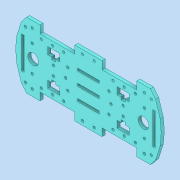
# Autodesk Inventor part: 底盘设计2.0
Saved by Autodesk Inventor 2019 (Build 230136000, 136)
## iProperties
Created: 2020-10-19
Part Number: 底盘设计2.0
Material: 乙缩醛树脂，白色
Document SubType Name: Modeling
Designer: Wang Hua
Density: 1.425 g/cm^3
Appearance: 平滑 - 白色
Author: Wang Hua
Autodesk Inventor part; units mm, degrees
ref_plane "YZ Plane" through (0, 0, 0) normal (1, 0, 0) x (0, 1, 0)
ref_plane "XZ Plane" through (0, 0, 0) normal (0, 1, 0) x (-1, 0, 0)
ref_plane "XY Plane" through (0, 0, 0) normal (0, 0, 1) x (1, 0, 0)
sketch "草图1" plane through (0, 0, 0) normal (0, 0, 1) x (1, 0, 0)
  line L0 (-80, -42.5) -> (-80, -32.5) construction
  line L1 (80, -42.5) -> (-80, 42.5) construction
  line L2 (-80, -42.5) -> (80, 42.5) construction
  line L3 (-17.5754, 32.5) -> (-62.5754, 32.5)
  line L4 (-62.5754, 32.5) -> (-62.5754, 42.5)
  line L5 (-17.5754, 42.5) -> (-17.5754, 32.5)
  line L6 (0, 0) -> (0, 68.1065) construction
  line L7 (0, 0) -> (-105.3921, 0) construction
  line L8 (17.5754, 32.5) -> (62.5754, 32.5)
  line L9 (62.5754, 32.5) -> (62.5754, 42.5)
  line L10 (17.5754, 42.5) -> (17.5754, 32.5)
  line L11 (-17.5754, -32.5) -> (-62.5754, -32.5)
  line L12 (-62.5754, -32.5) -> (-62.5754, -42.5)
  line L13 (-17.5754, -42.5) -> (-17.5754, -32.5)
  line L14 (62.5754, -32.5) -> (62.5754, -42.5)
  line L15 (17.5754, -32.5) -> (62.5754, -32.5)
  line L16 (17.5754, -42.5) -> (17.5754, -32.5)
  line L17 (-80, 42.5) -> (-62.5754, 42.5)
  line L18 (-17.5754, 42.5) -> (17.5754, 42.5)
  line L19 (62.5754, 42.5) -> (80, 42.5)
  line L20 (80, -42.5) -> (62.5754, -42.5)
  line L21 (17.5754, -42.5) -> (-17.5754, -42.5)
  line L22 (-62.5754, -42.5) -> (-80, -42.5)
  arc A0 (-92.6213, 15.4186) -> (-92.6213, -15.4186) centre (4.8977, 0) ccw
  line L23 (-80, 42.5) -> (-86.7375, 34.0532)
  line L24 (-86.7375, 34.0532) -> (-92.6213, 15.4186)
  line L25 (-80, -42.5) -> (-86.7375, -34.0532)
  line L26 (-86.7375, -34.0532) -> (-92.6213, -15.4186)
  arc A1 (92.6213, -15.4186) -> (92.6213, 15.4186) centre (-4.8977, 0) ccw
  line L27 (80, 42.5) -> (86.7375, 34.0532)
  line L28 (86.7375, 34.0532) -> (92.6213, 15.4186)
  line L29 (80, -42.5) -> (86.7375, -34.0532)
  line L30 (86.7375, -34.0532) -> (92.6213, -15.4186)
  line L31 (80, 42.5) -> (80, 32.5) construction
  circle A2 centre (-71.2877, 0) radius 7
  line L32 (-83.1946, -20.7208) -> (-86.3946, -20.7208)
  line L33 (-86.3946, -20.7208) -> (-86.3946, 20.7208)
  line L34 (-86.3946, 20.7208) -> (-83.1946, 20.7208)
  line L35 (-83.1946, 20.7208) -> (-83.1946, -20.7208)
  line L36 (-83.1946, -20.7208) -> (-86.3946, 20.7208) construction
  line L37 (-86.3946, -20.7208) -> (-83.1946, 20.7208) construction
  line L38 (-35.0754, 53.2522) -> (-35.0754, 15.4186) construction
  line L39 (-52.6567, 14.2921) -> (-52.6567, 23.3874)
  line L40 (-52.6567, 23.3874) -> (-36.8922, 23.3874)
  line L41 (-36.8922, 23.3874) -> (-36.8922, 14.2921)
  line L42 (-27.1931, 14.2921) -> (-42.9577, 23.3874) construction
  line L43 (-42.9577, 14.2921) -> (-27.1931, 23.3874) construction
  line L44 (-42.2559, 11.1975) -> (-47.2929, 11.1975)
  line L45 (-47.2929, 11.1975) -> (-47.2929, 14.2921)
  line L46 (-42.2559, 14.2921) -> (-42.2559, 11.1975)
  line L47 (-32.5569, 11.1975) -> (-37.5939, 17.3867) construction
  line L48 (-37.5939, 11.1975) -> (-32.5569, 17.3867) construction
  line L49 (-36.8922, 14.2921) -> (-42.2559, 14.2921)
  line L50 (-47.2929, 14.2921) -> (-52.6567, 14.2921)
  line L51 (-14.0581, 18.6186) -> (14.0581, 18.6186)
  line L52 (14.0581, 18.6186) -> (14.0581, 15.4186)
  line L53 (14.0581, 15.4186) -> (-14.0581, 15.4186)
  line L54 (-14.0581, 15.4186) -> (-14.0581, 18.6186)
  line L55 (14.0581, -1.6) -> (-14.0581, -1.6)
  line L56 (-14.0581, -1.6) -> (-14.0581, 1.6)
  line L57 (-14.0581, 1.6) -> (14.0581, 1.6)
  line L58 (14.0581, 1.6) -> (14.0581, -1.6)
  line L59 (14.0581, -1.6) -> (-14.0581, 1.6) construction
  line L60 (-14.0581, -1.6) -> (14.0581, 1.6) construction
  line L61 (-52.6567, -14.2921) -> (-52.6567, -23.3874)
  line L62 (-52.6567, -23.3874) -> (-36.8922, -23.3874)
  line L63 (-36.8922, -23.3874) -> (-36.8922, -14.2921)
  line L64 (-42.2559, -11.1975) -> (-47.2929, -11.1975)
  line L65 (-47.2929, -11.1975) -> (-47.2929, -14.2921)
  line L66 (-42.2559, -14.2921) -> (-42.2559, -11.1975)
  line L67 (-36.8922, -14.2921) -> (-42.2559, -14.2921)
  line L68 (-47.2929, -14.2921) -> (-52.6567, -14.2921)
  line L69 (-14.0581, -18.6186) -> (14.0581, -18.6186)
  line L70 (14.0581, -18.6186) -> (14.0581, -15.4186)
  line L71 (14.0581, -15.4186) -> (-14.0581, -15.4186)
  line L72 (-14.0581, -15.4186) -> (-14.0581, -18.6186)
  line L73 (80, -42.5) -> (80, -32.5) construction
  line L74 (52.6567, 14.2921) -> (52.6567, 23.3874)
  line L75 (52.6567, 23.3874) -> (36.8922, 23.3874)
  line L76 (36.8922, 23.3874) -> (36.8922, 14.2921)
  line L77 (42.2559, 11.1975) -> (47.2929, 11.1975)
  line L78 (47.2929, 11.1975) -> (47.2929, 14.2921)
  line L79 (42.2559, 14.2921) -> (42.2559, 11.1975)
  line L80 (36.8922, 14.2921) -> (42.2559, 14.2921)
  line L81 (47.2929, 14.2921) -> (52.6567, 14.2921)
  line L82 (36.8922, -23.3874) -> (36.8922, -14.2921)
  line L83 (52.6567, -23.3874) -> (36.8922, -23.3874)
  line L84 (52.6567, -14.2921) -> (52.6567, -23.3874)
  line L85 (47.2929, -14.2921) -> (52.6567, -14.2921)
  line L86 (47.2929, -11.1975) -> (47.2929, -14.2921)
  line L87 (42.2559, -11.1975) -> (47.2929, -11.1975)
  line L88 (42.2559, -14.2921) -> (42.2559, -11.1975)
  line L89 (36.8922, -14.2921) -> (42.2559, -14.2921)
  circle A3 centre (71.2877, 0) radius 7
  line L90 (83.1946, -20.7208) -> (86.3946, -20.7208)
  line L91 (86.3946, -20.7208) -> (86.3946, 20.7208)
  line L92 (86.3946, 20.7208) -> (83.1946, 20.7208)
  line L93 (83.1946, 20.7208) -> (83.1946, -20.7208)
  line L94 (86.3946, -20.7208) -> (83.1946, 20.7208) construction
  line L95 (0, 0) -> (51.2908, 0) construction
  point P0 (-84.7946, 0)
  point P1 (7.5, 37.2039)
  point P2 (-7.5, 37.2039)
  point P3 (-21.5, 37.1159)
  point P4 (21.5, 37.1159)
  point P5 (-35.0754, 18.8397)
  point P6 (-45.0754, 6.0335)
  point P7 (7.5, -37.2039)
  point P8 (-7.5, -37.2039)
  point P9 (-21.5, -37.1159)
  point P10 (21.5, -37.1159)
  point P11 (-45.0754, -6.0335)
  point P12 (-29.2838, 0)
  point P13 (-26.6075, 13)
  point P14 (-26.6075, -13)
  point P15 (45.0754, 6.0335)
  point P16 (45.0754, -6.0335)
  point P17 (29.2838, 0)
  point P18 (26.6075, 13)
  point P19 (26.6075, -13)
  point P20 (-81.3188, 31.1796)
  point P21 (-81.3188, -31.1796)
  point P22 (81.3188, 31.1796)
  point P23 (81.3188, -31.1796)
  point P24 (60.8153, 27.4236)
  point P25 (46.3153, 27.4236)
  point P26 (31.8153, 27.4236)
  point P27 (60.8153, -27.4236)
  point P28 (46.3153, -27.4236)
  point P29 (31.8153, -27.4236)
  point P30 (-60.8153, 27.4236)
  point P31 (-46.3153, 27.4236)
  point P32 (-31.8153, 27.4236)
  point P33 (-46.3153, -27.4236)
  point P34 (-60.8153, -27.4236)
  point P35 (-31.8153, -27.4236)
  point P36 (72.4718, 34.0532)
  point P37 (72.4718, 17.0686)
  point P38 (72.4718, -34.0532)
  point P39 (72.4718, -17.0686)
  point P40 (-72.4718, 34.0532)
  point P41 (-72.4718, 17.0686)
  point P42 (-72.4718, -17.0686)
  point P43 (-72.4718, -34.0532)
  point P44 (-40.0754, 32.5)
  point P45 (40.0754, 32.5)
  dimension "d0" = 160
  dimension "d1" = 85
  dimension "d2" = 10
  dimension "d3" = 45
  dimension "d4" = 14
  dimension "d5" = 3.2
  dimension "d6" = 7.5
  dimension "d7" = 14
  dimension "d8" = 17.5
  dimension "d9" = 3.2
  dimension "d10" = 3.2
  dimension "d11" = 13
  dimension "d16" = 14.5
  dimension "d17" = 14.5
  constraints: 192 end point, 68 symmetric about line, 21 parallel, 12 horizontal, 10 midpoint, 10 perpendicular, 7 point on line, 4 centre point, 4 point on circle, 2 vertical, 5 other
  measures "d0" distance of L2.end L1.end
  measures "d1" distance of L0.start L1.end
  measures "d2" distance of L12.start L12.end
  measures "d3" distance of L3.start L3.end
  measures "d4" diameter of A2
  measures "d5" distance of L34.end L33.end
  measures "d6" distance from line of point (7.5, 37.204) L6
  measures "d7" horizontal distance of point (21.5, 37.116) point (7.5, 37.204)
  measures "d8" distance between parallel lines of L5 L38
  measures "d9" distance of L53.end L51.start
  measures "d10" distance of L55.end L56.end
  measures "d11" distance from line of L7 point (-26.608, 13)
  measures "d16" distance of point (46.315, 27.424) point (60.815, 27.424)
  measures "d17" distance of point (31.815, 27.424) point (46.315, 27.424)
extrude "拉伸1" add sketch "草图1" along normal blind 4
hole "孔1" at (7.5, 37.2039, 0) at (-7.5, 37.2039, 0) at (-21.5, 37.1159, 0) at (21.5, 37.1159, 0) at (-45.0754, 6.0335, 0) at (21.5, -37.1159, 0) at (7.5, -37.2039, 0) at (-7.5, -37.2039, 0) at (-21.5, -37.1159, 0) at (-45.0754, -6.0335, 0) at (-29.2838, 0, 0) at (-26.6075, 13, 0) at (-26.6075, -13, 0) at (45.0754, 6.0335, 0) at (45.0754, -6.0335, 0) at (29.2838, 0, 0) at (26.6075, 13, 0) at (26.6075, -13, 0) at (-81.3188, 31.1796, 0) at (-81.3188, -31.1796, 0) at (81.3188, 31.1796, 0) at (81.3188, -31.1796, 0) at (60.8153, 27.4236, 0) at (46.3153, 27.4236, 0) at (31.8153, 27.4236, 0) at (46.3153, -27.4236, 0) at (60.8153, -27.4236, 0) at (31.8153, -27.4236, 0) at (-60.8153, 27.4236, 0) at (-46.3153, 27.4236, 0) at (-31.8153, 27.4236, 0) at (-60.8153, -27.4236, 0) at (-46.3153, -27.4236, 0) at (-31.8153, -27.4236, 0) at (72.4718, 34.0532, 0) at (72.4718, 17.0686, 0) at (72.4718, -17.0686, 0) at (72.4718, -34.0532, 0) at (-72.4718, 34.0532, 0) at (-72.4718, 17.0686, 0) at (-72.4718, -17.0686, 0) at (-72.4718, -34.0532, 0) direction (0, 0, 1) diameter 3.2 end through all
